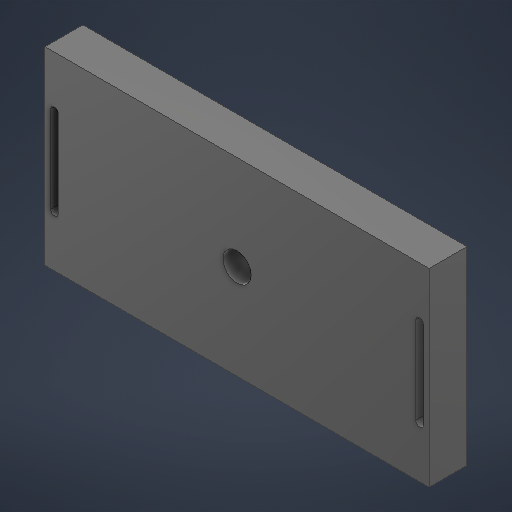
# Autodesk Inventor part: Part4
Saved by Autodesk Inventor 2026.2 (Build 302298010, 298A)
## iProperties
Created: 2026-03-02
Part Number: Part4
Material: Generic
Document SubType Name: Modeling
Designer: shahd
Density: 1 g/cm^3
Appearance: Default
Author: shahd
Autodesk Inventor part; units mm, degrees
ref_plane "YZ Plane" through (0, 0, 0) normal (1, 0, 0) x (0, 1, 0)
ref_plane "XZ Plane" through (0, 0, 0) normal (0, 1, 0) x (-1, 0, 0)
ref_plane "XY Plane" through (0, 0, 0) normal (0, 0, 1) x (1, 0, 0)
sketch "Sketch1" plane through (0, 0, 0) normal (0, 0, 1) x (1, 0, 0)
  line L0 (0, 0) -> (101.4, 0)
  line L1 (101.4, 0) -> (101.4, 50)
  line L2 (101.4, 50) -> (0, 50)
  line L3 (0, 50) -> (0, 0)
  circle A0 centre (50.7, 25) radius 3.75
  line L4 (2.5, 36.45) -> (2.5, 13.55) construction
  line L5 (1.45, 36.45) -> (1.45, 13.55)
  line L6 (3.55, 13.55) -> (3.55, 36.45)
  arc A1 (3.55, 36.45) -> (1.45, 36.45) centre (2.5, 36.45) ccw
  arc A2 (1.45, 13.55) -> (3.55, 13.55) centre (2.5, 13.55) ccw
  line L7 (101.4, 50) -> (101.4, 0)
  line L8 (98.9, 36.45) -> (98.9, 13.55) construction
  line L9 (99.95, 36.45) -> (99.95, 13.55)
  line L10 (97.85, 13.55) -> (97.85, 36.45)
  arc A3 (99.95, 36.45) -> (97.85, 36.45) centre (98.9, 36.45) ccw
  arc A4 (97.85, 13.55) -> (99.95, 13.55) centre (98.9, 13.55) ccw
  point P0 (2.5, 25)
  point P1 (2.5, 12.5)
  point P2 (2.5, 37.5)
  point P3 (98.9, 25)
  point P4 (98.9, 12.5)
  point P5 (98.9, 37.5)
  dimension "d2" = 101.4
  dimension "d3" = 50
  dimension "d23" = 7.5
  dimension "d24" = 25
  dimension "d25" = 50.7
  dimension "d26" = 2.1
  dimension "d28" = 25
  dimension "d29" = 25
  dimension "d31" = 2.5
  constraints: 26 end point, 10 point on circle, 5 centre point, 4 tangent, 3 parallel, 1 horizontal, 1 midpoint, 1 perpendicular, 1 vertical
  measures "d2" distance of L1.end L2.end
  measures "d3" distance of L0.end L1.end
  measures "d23" diameter of A0
  measures "d24" vertical distance of L0.start A0.centre
  measures "d25" horizontal distance of L0.start A0.centre
  measures "d26" diameter of A2
  measures "d28" vertical distance of L0.start point (2.5, 25)
  measures "d29" distance of point (2.5, 12.5) point (2.5, 37.5)
  measures "d31" horizontal distance of point (2.5, 25) L0.start
extrude "Extrusion1" add sketch "Sketch1" along normal mid plane 10
body "Solid1"
